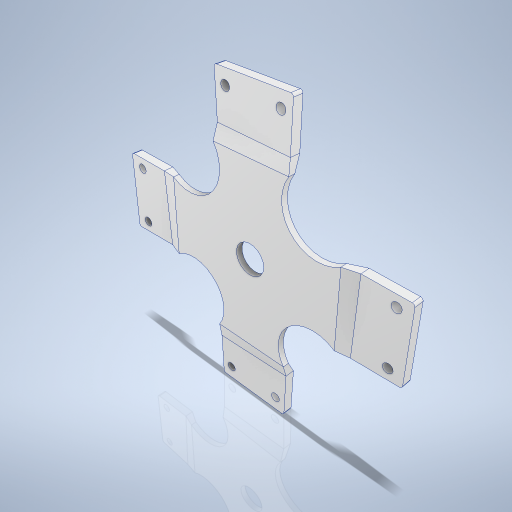
# Autodesk Inventor part: propeller
Saved by Autodesk Inventor 2024.2 (Build 282272000, 272)
## iProperties
Created: 2024-05-13
Part Number: propeller
Material: Aluminium 6061
Document SubType Name: Sheet Metal
Designer: Fabri
Density: 2.7 g/cm^3
Sheet Metal Rule: Standard_mm
Appearance: Aluminium - flach
Author: Fabri
Autodesk Inventor part; units mm, degrees
note: some values were not read from the file. Chosen so that the rebuilt part matches the saved one: direction of "Bohrung1".
ref_plane "YZ Plane" through (0, 0, 0) normal (1, 0, 0) x (0, 1, 0)
sketch "Skizze1" plane through (0, 0, 0) normal (0, 1, 0) x (-1, 0, 0)
  circle A0 centre (0, 0) radius 32
  dimension "d0" = 64
  measures "d0" diameter of A0
extrude "Grobblech1" add sketch "Skizze1" along normal mid plane 2
sketch "Skizze4" plane through (0, 1, 0) normal (0, 1, 0) x (1, 0, 0)
  circle A0 centre (0, 0) radius 32 projected
  line L0 (32, 0) -> (-32, 0) construction
  line L1 (0, 0) -> (-26.8083, -26.8083) construction
  circle A1 centre (0, 0) radius 32 projected
  line L2 (0, 0) -> (0, -36.5121) construction
  arc A2 (-12.7016, -29.3712) -> (-29.3712, -12.7016) centre (-22.6274, -22.6274) ccw
  line L3 (-12.7016, -29.3712) -> (12.7016, -29.3712)
  point P0 (12.7016, -29.3712)
  point P1 (-12.7016, -29.3712)
  point P2 (-12.7016, -29.3712)
  point P3 (-29.3712, -12.7016)
  dimension "d15" = 45
  dimension "d18" = 12
  constraints: 8 end point, 8 point on circle, 1 centre point, 1 horizontal, 1 midpoint, 1 perpendicular, 1 symmetric about line, 1 vertical
  measures "d15" angle of L0 L1
  measures "d18" radius of A2
extrude "Extrusion3" cut sketch "Skizze4" against normal up to surface (2 mm away) contours A2 A0 | A0 L3
pattern_circular "Runde Anordnung2" count 4 over 360 about axis through (0, -1, 0) along (0, 1, 0) of "Extrusion3"
sketch "Skizze5" plane through (0, 1, 0) normal (0, 1, 0) x (1, 0, 0)
  point P0 (0, 0)
  point P1 (0, 0)
  constraints: 1 coincident
hole "Bohrung1" at (0, 1, 0) direction (0, -1, 0) diameter 10 depth 2
ref_plane "Arbeitsebene1" through (0, 0, 49) normal (0, 0, 1) x (1, 0, 0)
ref_plane "Arbeitsebene2" through (0, 0, 34) normal (0, 0, 1) x (1, 0, 0)
sketch "Skizze6" plane through (0, 0, 34) normal (0, 0, 1) x (1, 0, 0)
  line L0 (0, 0) -> (-0.9271, 2.8532) construction
  line L1 (12.5, -0.4365) -> (-12.5, 0.4365)
  line L2 (-12.5, 0.4365) -> (-12.5, 3.4402)
  line L3 (-12.5, 3.4402) -> (12.6048, 2.5635)
  line L4 (12.6048, 2.5635) -> (12.5, -0.4365)
  point P0 (0, 0)
  dimension "d34" = 110
  dimension "d35" = 25
  dimension "d36" = 3
  constraints: 10 end point, 1 midpoint, 1 parallel, 1 perpendicular, 1 point on line
  measures "d34" angle of L0 L1
  measures "d35" horizontal distance of L1.end L1.start
  measures "d36" vertical distance of L3.end L1.start
sketch "Skizze7" plane through (-12.7016, -1, 29.3712) normal (0, 0, 1) x (1, 0, 0)
  line L0 (25.4033, 0) -> (0, 0) projected
  line L1 (25.4033, 2) -> (25.4033, 0) projected
  line L2 (0, 2) -> (25.4033, 2) projected
  line L3 (0, 0) -> (0, 2) projected
  point P0 (12.7016, 1)
loft "Erhebung1" add profiles "Skizze6" section 1 edges at (0, -1, 29.3712) (12.7016, 0, 29.3712) (0, 1, 29.3712) (-12.7016, 0, 29.3712)
sketch "Skizze8" plane through (0, 0, 49) normal (0, 0, 1) x (1, 0, 0)
  line L0 (0, 0) -> (0, -4.6524) construction
  line L1 (12.5, 0) -> (-12.5, 0)
  line L2 (12.5, 0) -> (12.5, 3)
  line L3 (12.5, 3) -> (-12.5, 3)
  line L4 (-12.5, 3) -> (-12.5, 0)
  point P0 (12.5, -0.4365)
  dimension "d41" = 90
  dimension "d42" = 25
  dimension "d43" = 3
  constraints: 10 end point, 2 parallel, 2 vertical, 1 midpoint
  measures "d41" angle of L0 L1
  measures "d42" distance of L1.start L1.end
  measures "d43" distance of L1.start L2.end
loft "Erhebung2" add profiles "Skizze8" section 1 edges at (0, 0, 34) (12.5524, 1.0635, 34) (0.0524, 3.0018, 34) (-12.5, 1.9383, 34)
pattern_circular "Runde Anordnung3" count 4 over 360 about axis through (0, -82.0984, 0) along (0, 1, 0) of "Erhebung1", "Erhebung2"
fillet "Rundung1" radius 0.8 2 edges at (49, 1.5, 12.5) (49, 1.5, -12.5)
fillet "Rundung2" radius 0.8 2 edges at (12.5, 1.5, -49) (-12.5, 1.5, -49)
fillet "Rundung3" radius 0.8 2 edges at (-49, 1.5, -12.5) (-49, 1.5, 12.5)
fillet "Rundung4" radius 0.8 2 edges at (-12.5, 1.5, 49) (12.5, 1.5, 49)
sketch "Skizze14" plane through (0, 1, 0) normal (0, 1, 0) x (1, 0, 0)
  line L0 (-34, -12.5) -> (-48.2, -12.5) projected
  line L1 (-49, -11.7) -> (-49, 11.7) projected
  line L2 (-34, 12.5) -> (-48.2, 12.5) projected
  point P0 (0, 0)
  point P1 (-44.5, -9)
  point P2 (-44.5, 9)
  dimension "d107" = 3.5
  dimension "d108" = 4.5
  dimension "d109" = 4.5
  dimension "d110" = 3.5
  measures "d107" distance from line of L0 point (-44.5, -9)
  measures "d108" distance from line of point (-44.5, -9) L1
  measures "d109" distance from line of point (-44.5, 9) L1
  measures "d110" distance from line of L2 point (-44.5, 9)
hole "Bohrung6" at (-44.5, 1, 9) at (-44.5, 1, -9) direction (0, -1, 0) diameter 3 end through all both
pattern_circular "Runde Anordnung4" count 4 over 360 about axis through (0, -82.0984, 0) along (0, 1, 0) of "Bohrung6"
equation "\"d29\" = Stärke"
equation "\"d116\" = Stärke"
equation "\"d1\" = Stärke"
equation "\"Biegeradius\" = Stärke"
equation "\"BreiteBiegungsfreistellung\" = Stärke"
equation "\"TiefeBiegungsfreistellung\" = 0.5 * Stärke"
equation "\"GrößeEckenfreistellung\" = 4 * Stärke"
equation "\"MinimalRest\" = 2 * Stärke"
equation "\"Übergangsradius\" = Biegeradius"
equation "\"JacobiRadiusGröße\" = Biegeradius"
equation "\"Abstandsgröße\" = Stärke"
equation "\"Stärke\" = 2"
